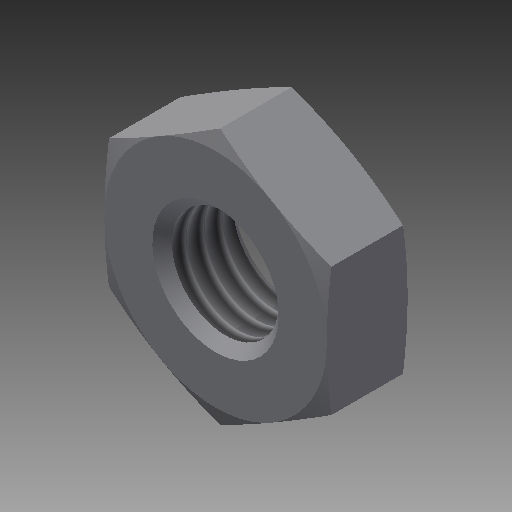
# Autodesk Inventor part: D-344
Saved by Autodesk Inventor 2019 (Build 230136000, 136)
## iProperties
Category: PARTsolutions
Company: BIMBA
Created: 2019-01-26
Part Number: D-344
Material: Generic
Catalog Web Link: www.cadenas.de
Description: Mounting Nut for Original Line Cylinders-
Vendor: BIMBA
Document SubType Name: Modeling
Designer: psadmin
Manufacturer: BIMBA
Mass: 0.34193 g
Surface Area: 3.8243 cm^2
Volume: 0.34193 cm^3
Density: 1 g/cm^3
Appearance: PSOLRGB-191-191-191
PSOL_IDENT_0: {$CADENAS_DATA\23d-libs\bimba\bimba\bimba_imperial\bimba_full_line\original_line_cylinders\accessori
PSOL_IDENT_1: es\mounting_nut.prj},187 {VTYP=3D},{NB=D-344},{LINA=D-344},{NN=Mounting Nut for Original Line Cylind
PSOL_IDENT_2: ers},{DATE=27.12.2018 09:32:42},{GEOMDATE=10.11.2011 00:00:00},{VERSION=},{LINEID=10},{WBVAR=MAT},{W
PSOL_IDENT_3: BNUMERIC=}  {NB=D-344},{LINA=D-344},{KT=DUMMY},{PN=D-344},{PN1=D-344},{C=1/4-28},{TH=UNF},{MAT=},{MA
PSOL_IDENT_4: T1='','Zinc-Plated Carbon Steel', '-SS', 'Stainless Steel'},{A=0.44},{A1=0.44000000},{B=0.16},{B1=0.
PSOL_IDENT_5: 16000000},{NDM=0.25000000},{PITCH=0.0357},{DIA=-},{DIA2=-},{DIA3=-},{DIA1=0},{DIA4=0.00000000},{DIA5=
PSOL_IDENT_6: 0.00000000},{T=-},{T2=-},{T3=-},{T1=0},{T4=0.00000000},{T5=0.00000000},{COLOR=0.75,0.75,0.75,0.00},{
PSOL_IDENT_7: TT=0.05000000},{TO=0.15000000},{PRA=1}
NN: Mounting Nut for Original Line Cylinders
NB: D-344
NBSYN: $PN.
LINA: D-344
PN: D-344
C: 1/4-28
MAT: Zinc-Plated Carbon Steel
A: 0.44
B: 0.16
DIA: -
T: -
SUPPLIER: BIMBA
ARTICLENO: D-344
BOMINFO: D-344
CREATOR: CADENAS GmbH
Title: D-344
Author: Cadenas PARTsolutions
Autodesk Inventor part; units mm, degrees
ref_plane "YZ Plane" through (0, 0, 0) normal (1, 0, 0) x (0, 1, 0)
ref_plane "XZ Plane" through (0, 0, 0) normal (0, 1, 0) x (-1, 0, 0)
ref_plane "XY Plane" through (0, 0, 0) normal (0, 0, 1) x (1, 0, 0)
sketch "Sketch_8" plane through (0, 0, 0) normal (1, 0, 0) x (0, 1, 0)
  line L0 (0, -4.064) -> (0, 0)
  line L1 (0, 0) -> (5.588, 0)
  line L2 (5.588, 0) -> (6.7056, -0.2995)
  line L3 (6.7056, -0.2995) -> (6.7056, -3.7645)
  line L4 (6.7056, -3.7645) -> (5.588, -4.064)
  line L5 (5.588, -4.064) -> (0, -4.064)
  line L6 (0, -4.064) -> (0, 0)
  constraints: 14 end point
sketch "Sketch_10" plane through (0, 0, 0) normal (0, 0, 1) x (1, 0, 0)
  line L0 (-11.176, -11.176) -> (11.176, -11.176)
  line L1 (11.176, -11.176) -> (11.176, 11.176)
  line L2 (11.176, 11.176) -> (-11.176, 11.176)
  line L3 (-11.176, 11.176) -> (-11.176, -11.176)
  line L4 (-5.588, -3.2262) -> (0, -6.4525)
  line L5 (0, -6.4525) -> (5.588, -3.2262)
  line L6 (5.588, -3.2262) -> (5.588, 3.2262)
  line L7 (5.588, 3.2262) -> (0, 6.4525)
  line L8 (0, 6.4525) -> (-5.588, 3.2262)
  line L9 (-5.588, 3.2262) -> (-5.588, -3.2262)
  constraints: 20 end point
revolve "Revolution1" add sketch "Sketch_8" angle 360 about axis through (0, 0, -4.064) along (0, 0, -1)
extrude "Extrusion1" cut sketch "Sketch_10" against normal blind 4.064
sketch "Sketch_11" plane through (0, 0, 0) normal (1, 0, 0) x (0, 1, 0)
  line L0 (0, -4.064) -> (0, 0)
  line L1 (0, 0) -> (3.175, 0)
  line L2 (3.175, 0) -> (2.6835, -0.4915)
  line L3 (2.6835, -0.4915) -> (2.6835, -3.5725)
  line L4 (2.6835, -3.5725) -> (3.175, -4.064)
  line L5 (3.175, -4.064) -> (0, -4.064)
  line L6 (0, -4.064) -> (0, 0)
  constraints: 14 end point
revolve "Revolution2" cut sketch "Sketch_11" angle 360 about axis through (0, 0, -4.064) along (0, 0, -1)
thread "Thread1" size "1/4-28 UNF" class "2B" standard "ANSI Unified Screw Threads" full length
ref_plane "NUT_XY" through (0, 0, 0) normal (0, 0, 1) x (1, 0, 0)
ref_plane "NUT_YZ" through (0, 0, 0) normal (1, 0, 0) x (0, 1, 0)
ref_plane "NUT_ZX" through (0, 0, 0) normal (0, 1, 0) x (0, 0, 1)
ref_plane "a1_XY" through (-5.588, 5.588, 0) normal (0, 0, 1) x (1, 0, 0)
ref_plane "a1_YZ" through (-5.588, 5.588, 0) normal (1, 0, 0) x (0, 1, 0)
ref_plane "a1_ZX" through (-5.588, 5.588, 0) normal (0, 1, 0) x (0, 0, 1)
ref_plane "a2_XY" through (5.588, 5.588, 0) normal (0, 0, 1) x (1, 0, 0)
ref_plane "a2_YZ" through (5.588, 5.588, 0) normal (1, 0, 0) x (0, 1, 0)
ref_plane "a2_ZX" through (5.588, 5.588, 0) normal (0, 1, 0) x (0, 0, 1)
ref_plane "b1_XY" through (0, 5.588, 0) normal (1, 0, 0) x (0, 0, -1)
ref_plane "b1_YZ" through (0, 5.588, 0) normal (0, 0, -1) x (0, 1, 0)
ref_plane "b1_ZX" through (0, 5.588, 0) normal (0, 1, 0) x (1, 0, 0)
ref_plane "b2_XY" through (0, 5.588, -4.064) normal (1, 0, 0) x (0, 0, -1)
ref_plane "b2_YZ" through (0, 5.588, -4.064) normal (0, 0, -1) x (0, 1, 0)
ref_plane "b2_ZX" through (0, 5.588, -4.064) normal (0, 1, 0) x (1, 0, 0)
ref_plane "e_XY" through (0, 0, -4.064) normal (1, 0, 0) x (0, 0, -1)
ref_plane "e_YZ" through (0, 0, -4.064) normal (0, 0, -1) x (0, 1, 0)
ref_plane "e_ZX" through (0, 0, -4.064) normal (0, 1, 0) x (1, 0, 0)
ref_plane "ol1_XY" through (0, 0, -5.588) normal (0, 1, 0) x (1, 0, 0)
ref_plane "ol1_YZ" through (0, 0, -5.588) normal (1, 0, 0) x (0, 0, -1)
ref_plane "ol1_ZX" through (0, 0, -5.588) normal (0, 0, -1) x (0, 1, 0)
ref_plane "ol2_XY" through (4.064, 0, -5.588) normal (0, 1, 0) x (1, 0, 0)
ref_plane "ol2_YZ" through (4.064, 0, -5.588) normal (1, 0, 0) x (0, 0, -1)
ref_plane "ol2_ZX" through (4.064, 0, -5.588) normal (0, 0, -1) x (0, 1, 0)
ref_plane "th1_XY" through (0, 3.175, -4.064) normal (1, 0, 0) x (0, 0, -1)
ref_plane "th1_YZ" through (0, 3.175, -4.064) normal (0, 0, -1) x (0, 1, 0)
ref_plane "th1_ZX" through (0, 3.175, -4.064) normal (0, 1, 0) x (1, 0, 0)
ref_plane "th2_XY" through (0, -3.175, -4.064) normal (1, 0, 0) x (0, 0, -1)
ref_plane "th2_YZ" through (0, -3.175, -4.064) normal (0, 0, -1) x (0, 1, 0)
ref_plane "th2_ZX" through (0, -3.175, -4.064) normal (0, 1, 0) x (1, 0, 0)
body "Solid1"
